Autodesk Fusion 360 part; units mm, degrees
(part 2 of 3)
  line L366 (210.5589, 31.2011) -> (210.5337, 34.6652)
  line L367 (213.9873, 40.7539) -> (210.9748, 42.464)
  line L368 (204.5338, 34.6214) -> (204.559, 31.1574)
  line L369 (201.0129, 37.1927) -> (204.0254, 35.4826)
  line L370 (210.9748, 42.464) -> (207.9875, 40.7102)
  line L371 (200.9877, 40.6567) -> (201.0129, 37.1927)
  line L372 (214.5714, 29.5007) -> (217.5587, 31.2545)
  line L373 (211.5336, 34.6749) -> (211.5588, 31.2108)
  line L374 (214.5209, 36.4287) -> (211.5336, 34.6749)
  line L375 (206.9875, 40.7005) -> (203.975, 42.4106)
  line L376 (207.5716, 29.4473) -> (210.5589, 31.2011)
  line L377 (210.5337, 34.6652) -> (207.5211, 36.3753)
  line L378 (207.9875, 40.7102) -> (208.0127, 37.2461)
  line L379 (204.0254, 35.4826) -> (207.0127, 37.2364)
  line L380 (211.5588, 31.2108) -> (214.5714, 29.5007)
  line L381 (207.5211, 36.3753) -> (204.5338, 34.6214)
  line L382 (208.0127, 37.2461) -> (211.0252, 35.536)
  line L383 (211.0252, 35.536) -> (214.0125, 37.2898)
  line L384 (207.0127, 37.2364) -> (206.9875, 40.7005)
  line L385 (203.975, 42.4106) -> (200.9877, 40.6567)
  line L386 (204.559, 31.1574) -> (207.5716, 29.4473)
  line L387 (214.0125, 37.2898) -> (213.9873, 40.7539)
  line L388 (217.5587, 31.2545) -> (217.5335, 34.7186)
  line L389 (217.5335, 34.7186) -> (214.5209, 36.4287)
  line L390 (224.5589, 31.2011) -> (224.5337, 34.6652)
  line L391 (227.9873, 40.7539) -> (224.9748, 42.464)
  line L392 (218.5338, 34.6214) -> (218.559, 31.1574)
  line L393 (215.0129, 37.1927) -> (218.0254, 35.4826)
  line L394 (224.9748, 42.464) -> (221.9875, 40.7102)
  line L395 (214.9877, 40.6567) -> (215.0129, 37.1927)
  line L396 (228.5714, 29.5007) -> (231.5587, 31.2545)
  line L397 (225.5336, 34.6749) -> (225.5588, 31.2108)
  line L398 (228.5209, 36.4287) -> (225.5336, 34.6749)
  line L399 (220.9875, 40.7005) -> (217.975, 42.4106)
  line L400 (221.5716, 29.4473) -> (224.5589, 31.2011)
  line L401 (224.5337, 34.6652) -> (221.5211, 36.3753)
  line L402 (221.9875, 40.7102) -> (222.0127, 37.2461)
  line L403 (218.0254, 35.4826) -> (221.0127, 37.2364)
  line L404 (225.5588, 31.2108) -> (228.5714, 29.5007)
  line L405 (221.5211, 36.3753) -> (218.5338, 34.6214)
  line L406 (222.0127, 37.2461) -> (225.0252, 35.536)
  line L407 (225.0252, 35.536) -> (228.0125, 37.2898)
  line L408 (221.0127, 37.2364) -> (220.9875, 40.7005)
  line L409 (217.975, 42.4106) -> (214.9877, 40.6567)
  line L410 (218.559, 31.1574) -> (221.5716, 29.4473)
  line L411 (228.0125, 37.2898) -> (227.9873, 40.7539)
  line L412 (231.5587, 31.2545) -> (231.5335, 34.7186)
  line L413 (231.5335, 34.7186) -> (228.5209, 36.4287)
  line L414 (140.5589, 43.2011) -> (140.5337, 46.6652)
  line L415 (143.9873, 52.7539) -> (140.9748, 54.464)
  line L416 (134.5338, 46.6214) -> (134.559, 43.1574)
  line L417 (131.0129, 49.1927) -> (134.0254, 47.4826)
  line L418 (140.9748, 54.464) -> (137.9875, 52.7102)
  line L419 (130.9877, 52.6567) -> (131.0129, 49.1927)
  line L420 (144.5714, 41.5007) -> (147.5587, 43.2545)
  line L421 (141.5336, 46.6749) -> (141.5588, 43.2108)
  line L422 (144.5209, 48.4287) -> (141.5336, 46.6749)
  line L423 (136.9875, 52.7005) -> (133.975, 54.4106)
  line L424 (137.5716, 41.4473) -> (140.5589, 43.2011)
  line L425 (140.5337, 46.6652) -> (137.5211, 48.3753)
  line L426 (137.9875, 52.7102) -> (138.0127, 49.2461)
  line L427 (134.0254, 47.4826) -> (137.0127, 49.2364)
  line L428 (141.5588, 43.2108) -> (144.5714, 41.5007)
  line L429 (137.5211, 48.3753) -> (134.5338, 46.6214)
  line L430 (138.0127, 49.2461) -> (141.0252, 47.536)
  line L431 (141.0252, 47.536) -> (144.0125, 49.2898)
  line L432 (137.0127, 49.2364) -> (136.9875, 52.7005)
  line L433 (133.975, 54.4106) -> (130.9877, 52.6567)
  line L434 (134.559, 43.1574) -> (137.5716, 41.4473)
  line L435 (144.0125, 49.2898) -> (143.9873, 52.7539)
  line L436 (147.5587, 43.2545) -> (147.5335, 46.7186)
  line L437 (147.5335, 46.7186) -> (144.5209, 48.4287)
  line L438 (154.5589, 43.2011) -> (154.5337, 46.6652)
  line L439 (157.9873, 52.7539) -> (154.9748, 54.464)
  line L440 (148.5338, 46.6214) -> (148.559, 43.1574)
  line L441 (145.0129, 49.1927) -> (148.0254, 47.4826)
  line L442 (154.9748, 54.464) -> (151.9875, 52.7102)
  line L443 (144.9877, 52.6567) -> (145.0129, 49.1927)
  line L444 (158.5714, 41.5007) -> (161.5587, 43.2545)
  line L445 (155.5336, 46.6749) -> (155.5588, 43.2108)
  line L446 (158.5209, 48.4287) -> (155.5336, 46.6749)
  line L447 (150.9875, 52.7005) -> (147.975, 54.4106)
  line L448 (151.5716, 41.4473) -> (154.5589, 43.2011)
  line L449 (154.5337, 46.6652) -> (151.5211, 48.3753)
  line L450 (151.9875, 52.7102) -> (152.0127, 49.2461)
  line L451 (148.0254, 47.4826) -> (151.0127, 49.2364)
  line L452 (155.5588, 43.2108) -> (158.5714, 41.5007)
  line L453 (151.5211, 48.3753) -> (148.5338, 46.6214)
  line L454 (152.0127, 49.2461) -> (155.0252, 47.536)
  line L455 (155.0252, 47.536) -> (158.0125, 49.2898)
  line L456 (151.0127, 49.2364) -> (150.9875, 52.7005)
  line L457 (147.975, 54.4106) -> (144.9877, 52.6567)
  line L458 (148.559, 43.1574) -> (151.5716, 41.4473)
  line L459 (158.0125, 49.2898) -> (157.9873, 52.7539)
  line L460 (161.5587, 43.2545) -> (161.5335, 46.7186)
  line L461 (161.5335, 46.7186) -> (158.5209, 48.4287)
  line L462 (168.5589, 43.2011) -> (168.5337, 46.6652)
  line L463 (171.9873, 52.7539) -> (168.9748, 54.464)
  line L464 (162.5338, 46.6214) -> (162.559, 43.1574)
  line L465 (159.0129, 49.1927) -> (162.0254, 47.4826)
  line L466 (168.9748, 54.464) -> (165.9875, 52.7102)
  line L467 (158.9877, 52.6567) -> (159.0129, 49.1927)
  line L468 (172.5714, 41.5007) -> (175.5587, 43.2545)
  line L469 (169.5336, 46.6749) -> (169.5588, 43.2108)
  line L470 (172.5209, 48.4287) -> (169.5336, 46.6749)
  line L471 (164.9875, 52.7005) -> (161.975, 54.4106)
  line L472 (165.5716, 41.4473) -> (168.5589, 43.2011)
  line L473 (168.5337, 46.6652) -> (165.5211, 48.3753)
  line L474 (165.9875, 52.7102) -> (166.0127, 49.2461)
  line L475 (162.0254, 47.4826) -> (165.0127, 49.2364)
  line L476 (169.5588, 43.2108) -> (172.5714, 41.5007)
  line L477 (165.5211, 48.3753) -> (162.5338, 46.6214)
  line L478 (166.0127, 49.2461) -> (169.0252, 47.536)
  line L479 (169.0252, 47.536) -> (172.0125, 49.2898)
  line L480 (165.0127, 49.2364) -> (164.9875, 52.7005)
  line L481 (161.975, 54.4106) -> (158.9877, 52.6567)
  line L482 (162.559, 43.1574) -> (165.5716, 41.4473)
  line L483 (172.0125, 49.2898) -> (171.9873, 52.7539)
  line L484 (175.5587, 43.2545) -> (175.5335, 46.7186)
  line L485 (175.5335, 46.7186) -> (172.5209, 48.4287)
  line L486 (182.5589, 43.2011) -> (182.5337, 46.6652)
  line L487 (185.9873, 52.7539) -> (182.9748, 54.464)
  line L488 (176.5338, 46.6214) -> (176.559, 43.1574)
  line L489 (173.0129, 49.1927) -> (176.0254, 47.4826)
  line L490 (182.9748, 54.464) -> (179.9875, 52.7102)
  line L491 (172.9877, 52.6567) -> (173.0129, 49.1927)
  line L492 (186.5714, 41.5007) -> (189.5587, 43.2545)
  line L493 (183.5336, 46.6749) -> (183.5588, 43.2108)
  line L494 (186.5209, 48.4287) -> (183.5336, 46.6749)
  line L495 (178.9875, 52.7005) -> (175.975, 54.4106)
  line L496 (179.5716, 41.4473) -> (182.5589, 43.2011)
  line L497 (182.5337, 46.6652) -> (179.5211, 48.3753)
  line L498 (179.9875, 52.7102) -> (180.0127, 49.2461)
  line L499 (176.0254, 47.4826) -> (179.0127, 49.2364)
  line L500 (183.5588, 43.2108) -> (186.5714, 41.5007)
  line L501 (179.5211, 48.3753) -> (176.5338, 46.6214)
  line L502 (180.0127, 49.2461) -> (183.0252, 47.536)
  line L503 (183.0252, 47.536) -> (186.0125, 49.2898)
  line L504 (179.0127, 49.2364) -> (178.9875, 52.7005)
  line L505 (175.975, 54.4106) -> (172.9877, 52.6567)
  line L506 (176.559, 43.1574) -> (179.5716, 41.4473)
  line L507 (186.0125, 49.2898) -> (185.9873, 52.7539)
  line L508 (189.5587, 43.2545) -> (189.5335, 46.7186)
  line L509 (189.5335, 46.7186) -> (186.5209, 48.4287)
  line L510 (196.5589, 43.2011) -> (196.5337, 46.6652)
  line L511 (199.9873, 52.7539) -> (196.9748, 54.464)
  line L512 (190.5338, 46.6214) -> (190.559, 43.1574)
  line L513 (187.0129, 49.1927) -> (190.0254, 47.4826)
  line L514 (196.9748, 54.464) -> (193.9875, 52.7102)
  line L515 (186.9877, 52.6567) -> (187.0129, 49.1927)
  line L516 (200.5714, 41.5007) -> (203.5587, 43.2545)
  line L517 (197.5336, 46.6749) -> (197.5588, 43.2108)
  line L518 (200.5209, 48.4287) -> (197.5336, 46.6749)
  line L519 (192.9875, 52.7005) -> (189.975, 54.4106)
  line L520 (193.5716, 41.4473) -> (196.5589, 43.2011)
  line L521 (196.5337, 46.6652) -> (193.5211, 48.3753)
  line L522 (193.9875, 52.7102) -> (194.0127, 49.2461)
  line L523 (190.0254, 47.4826) -> (193.0127, 49.2364)
  line L524 (197.5588, 43.2108) -> (200.5714, 41.5007)
  line L525 (193.5211, 48.3753) -> (190.5338, 46.6214)
  line L526 (194.0127, 49.2461) -> (197.0252, 47.536)
  line L527 (197.0252, 47.536) -> (200.0125, 49.2898)
  line L528 (193.0127, 49.2364) -> (192.9875, 52.7005)
  line L529 (189.975, 54.4106) -> (186.9877, 52.6567)
  line L530 (190.559, 43.1574) -> (193.5716, 41.4473)
  line L531 (200.0125, 49.2898) -> (199.9873, 52.7539)
  line L532 (203.5587, 43.2545) -> (203.5335, 46.7186)
  line L533 (203.5335, 46.7186) -> (200.5209, 48.4287)
  line L534 (210.5589, 43.2011) -> (210.5337, 46.6652)
  line L535 (213.9873, 52.7539) -> (210.9748, 54.464)
  line L536 (204.5338, 46.6214) -> (204.559, 43.1574)
  line L537 (201.0129, 49.1927) -> (204.0254, 47.4826)
  line L538 (210.9748, 54.464) -> (207.9875, 52.7102)
  line L539 (200.9877, 52.6567) -> (201.0129, 49.1927)
  line L540 (214.5714, 41.5007) -> (217.5587, 43.2545)
  line L541 (211.5336, 46.6749) -> (211.5588, 43.2108)
  line L542 (214.5209, 48.4287) -> (211.5336, 46.6749)
  line L543 (206.9875, 52.7005) -> (203.975, 54.4106)
  line L544 (207.5716, 41.4473) -> (210.5589, 43.2011)
  line L545 (210.5337, 46.6652) -> (207.5211, 48.3753)
  line L546 (207.9875, 52.7102) -> (208.0127, 49.2461)
  line L547 (204.0254, 47.4826) -> (207.0127, 49.2364)
  line L548 (211.5588, 43.2108) -> (214.5714, 41.5007)
  line L549 (207.5211, 48.3753) -> (204.5338, 46.6214)
  line L550 (208.0127, 49.2461) -> (211.0252, 47.536)
  line L551 (211.0252, 47.536) -> (214.0125, 49.2898)
  line L552 (207.0127, 49.2364) -> (206.9875, 52.7005)
  line L553 (203.975, 54.4106) -> (200.9877, 52.6567)
  line L554 (204.559, 43.1574) -> (207.5716, 41.4473)
  line L555 (214.0125, 49.2898) -> (213.9873, 52.7539)
  line L556 (217.5587, 43.2545) -> (217.5335, 46.7186)
  line L557 (217.5335, 46.7186) -> (214.5209, 48.4287)
  line L558 (224.5589, 43.2011) -> (224.5337, 46.6652)
  line L559 (227.9873, 52.7539) -> (224.9748, 54.464)
  line L560 (218.5338, 46.6214) -> (218.559, 43.1574)
  line L561 (215.0129, 49.1927) -> (218.0254, 47.4826)
  line L562 (224.9748, 54.464) -> (221.9875, 52.7102)
  line L563 (214.9877, 52.6567) -> (215.0129, 49.1927)
  line L564 (228.5714, 41.5007) -> (231.5587, 43.2545)
  line L565 (225.5336, 46.6749) -> (225.5588, 43.2108)
  line L566 (228.5209, 48.4287) -> (225.5336, 46.6749)
  line L567 (220.9875, 52.7005) -> (217.975, 54.4106)
  line L568 (221.5716, 41.4473) -> (224.5589, 43.2011)
  line L569 (224.5337, 46.6652) -> (221.5211, 48.3753)
  line L570 (221.9875, 52.7102) -> (222.0127, 49.2461)
  line L571 (218.0254, 47.4826) -> (221.0127, 49.2364)
  line L572 (225.5588, 43.2108) -> (228.5714, 41.5007)
  line L573 (221.5211, 48.3753) -> (218.5338, 46.6214)
  line L574 (222.0127, 49.2461) -> (225.0252, 47.536)
  line L575 (225.0252, 47.536) -> (228.0125, 49.2898)
  line L576 (221.0127, 49.2364) -> (220.9875, 52.7005)
  line L577 (217.975, 54.4106) -> (214.9877, 52.6567)
  line L578 (218.559, 43.1574) -> (221.5716, 41.4473)
  line L579 (228.0125, 49.2898) -> (227.9873, 52.7539)
  line L580 (231.5587, 43.2545) -> (231.5335, 46.7186)
  line L581 (231.5335, 46.7186) -> (228.5209, 48.4287)
  line L582 (140.5589, 55.2011) -> (140.5337, 58.6652)
  line L583 (143.9873, 64.7539) -> (140.9748, 66.464)
  line L584 (134.5338, 58.6214) -> (134.559, 55.1574)
  line L585 (131.0129, 61.1927) -> (134.0254, 59.4826)
  line L586 (140.9748, 66.464) -> (137.9875, 64.7102)
  line L587 (130.9877, 64.6567) -> (131.0129, 61.1927)
  line L588 (144.5714, 53.5007) -> (147.5587, 55.2545)
  line L589 (141.5336, 58.6749) -> (141.5588, 55.2108)
  line L590 (144.5209, 60.4287) -> (141.5336, 58.6749)
  line L591 (136.9875, 64.7005) -> (133.975, 66.4106)
  line L592 (137.5716, 53.4473) -> (140.5589, 55.2011)
  line L593 (140.5337, 58.6652) -> (137.5211, 60.3753)
  line L594 (137.9875, 64.7102) -> (138.0127, 61.2461)
  line L595 (134.0254, 59.4826) -> (137.0127, 61.2364)
  line L596 (141.5588, 55.2108) -> (144.5714, 53.5007)
  line L597 (137.5211, 60.3753) -> (134.5338, 58.6214)
  line L598 (138.0127, 61.2461) -> (141.0252, 59.536)
  line L599 (141.0252, 59.536) -> (144.0125, 61.2898)
  line L600 (137.0127, 61.2364) -> (136.9875, 64.7005)
  line L601 (133.975, 66.4106) -> (130.9877, 64.6567)
  line L602 (134.559, 55.1574) -> (137.5716, 53.4473)
  line L603 (144.0125, 61.2898) -> (143.9873, 64.7539)
  line L604 (147.5587, 55.2545) -> (147.5335, 58.7186)
  line L605 (147.5335, 58.7186) -> (144.5209, 60.4287)
  line L606 (154.5589, 55.2011) -> (154.5337, 58.6652)
  line L607 (157.9873, 64.7539) -> (154.9748, 66.464)
  line L608 (148.5338, 58.6214) -> (148.559, 55.1574)
  line L609 (145.0129, 61.1927) -> (148.0254, 59.4826)
  line L610 (154.9748, 66.464) -> (151.9875, 64.7102)
  line L611 (144.9877, 64.6567) -> (145.0129, 61.1927)
  line L612 (158.5714, 53.5007) -> (161.5587, 55.2545)
  line L613 (155.5336, 58.6749) -> (155.5588, 55.2108)
  line L614 (158.5209, 60.4287) -> (155.5336, 58.6749)
  line L615 (150.9875, 64.7005) -> (147.975, 66.4106)
  line L616 (151.5716, 53.4473) -> (154.5589, 55.2011)
  line L617 (154.5337, 58.6652) -> (151.5211, 60.3753)
  line L618 (151.9875, 64.7102) -> (152.0127, 61.2461)
  line L619 (148.0254, 59.4826) -> (151.0127, 61.2364)
  line L620 (155.5588, 55.2108) -> (158.5714, 53.5007)
  line L621 (151.5211, 60.3753) -> (148.5338, 58.6214)
  line L622 (152.0127, 61.2461) -> (155.0252, 59.536)
  line L623 (155.0252, 59.536) -> (158.0125, 61.2898)
  line L624 (151.0127, 61.2364) -> (150.9875, 64.7005)
  line L625 (147.975, 66.4106) -> (144.9877, 64.6567)
  line L626 (148.559, 55.1574) -> (151.5716, 53.4473)
  line L627 (158.0125, 61.2898) -> (157.9873, 64.7539)
  line L628 (161.5587, 55.2545) -> (161.5335, 58.7186)
  line L629 (161.5335, 58.7186) -> (158.5209, 60.4287)
  line L630 (168.5589, 55.2011) -> (168.5337, 58.6652)
  line L631 (171.9873, 64.7539) -> (168.9748, 66.464)
  line L632 (162.5338, 58.6214) -> (162.559, 55.1574)
  line L633 (159.0129, 61.1927) -> (162.0254, 59.4826)
  line L634 (168.9748, 66.464) -> (165.9875, 64.7102)
  line L635 (158.9877, 64.6567) -> (159.0129, 61.1927)
  line L636 (172.5714, 53.5007) -> (175.5587, 55.2545)
  line L637 (169.5336, 58.6749) -> (169.5588, 55.2108)
  line L638 (172.5209, 60.4287) -> (169.5336, 58.6749)
  line L639 (164.9875, 64.7005) -> (161.975, 66.4106)
  line L640 (165.5716, 53.4473) -> (168.5589, 55.2011)
  line L641 (168.5337, 58.6652) -> (165.5211, 60.3753)
  line L642 (165.9875, 64.7102) -> (166.0127, 61.2461)
  line L643 (162.0254, 59.4826) -> (165.0127, 61.2364)
  line L644 (169.5588, 55.2108) -> (172.5714, 53.5007)
  line L645 (165.5211, 60.3753) -> (162.5338, 58.6214)
  line L646 (166.0127, 61.2461) -> (169.0252, 59.536)
  line L647 (169.0252, 59.536) -> (172.0125, 61.2898)
  line L648 (165.0127, 61.2364) -> (164.9875, 64.7005)
  line L649 (161.975, 66.4106) -> (158.9877, 64.6567)
  line L650 (162.559, 55.1574) -> (165.5716, 53.4473)
  line L651 (172.0125, 61.2898) -> (171.9873, 64.7539)
  line L652 (175.5587, 55.2545) -> (175.5335, 58.7186)
  line L653 (175.5335, 58.7186) -> (172.5209, 60.4287)
  line L654 (196.5589, 55.2011) -> (196.5337, 58.6652)
  line L655 (199.9873, 64.7539) -> (196.9748, 66.464)
  line L656 (190.5338, 58.6214) -> (190.559, 55.1574)
  line L657 (187.0129, 61.1927) -> (190.0254, 59.4826)
  line L658 (196.9748, 66.464) -> (193.9875, 64.7102)
  line L659 (186.9877, 64.6567) -> (187.0129, 61.1927)
  line L660 (200.5714, 53.5007) -> (203.5587, 55.2545)
  line L661 (197.5336, 58.6749) -> (197.5588, 55.2108)
  line L662 (200.5209, 60.4287) -> (197.5336, 58.6749)
  line L663 (192.9875, 64.7005) -> (189.975, 66.4106)
  line L664 (193.5716, 53.4473) -> (196.5589, 55.2011)
  line L665 (196.5337, 58.6652) -> (193.5211, 60.3753)
  line L666 (193.9875, 64.7102) -> (194.0127, 61.2461)
  line L667 (190.0254, 59.4826) -> (193.0127, 61.2364)
  line L668 (197.5588, 55.2108) -> (200.5714, 53.5007)
  line L669 (193.5211, 60.3753) -> (190.5338, 58.6214)
  line L670 (194.0127, 61.2461) -> (197.0252, 59.536)
  line L671 (197.0252, 59.536) -> (200.0125, 61.2898)
  line L672 (193.0127, 61.2364) -> (192.9875, 64.7005)
  line L673 (189.975, 66.4106) -> (186.9877, 64.6567)
  line L674 (190.559, 55.1574) -> (193.5716, 53.4473)
  line L675 (200.0125, 61.2898) -> (199.9873, 64.7539)
  line L676 (203.5587, 55.2545) -> (203.5335, 58.7186)
  line L677 (203.5335, 58.7186) -> (200.5209, 60.4287)
  line L678 (210.5589, 55.2011) -> (210.5337, 58.6652)
  line L679 (213.9873, 64.7539) -> (210.9748, 66.464)
  line L680 (204.5338, 58.6214) -> (204.559, 55.1574)
  line L681 (201.0129, 61.1927) -> (204.0254, 59.4826)
  line L682 (210.9748, 66.464) -> (207.9875, 64.7102)
  line L683 (200.9877, 64.6567) -> (201.0129, 61.1927)
  line L684 (214.5714, 53.5007) -> (217.5587, 55.2545)
  line L685 (211.5336, 58.6749) -> (211.5588, 55.2108)
  line L686 (214.5209, 60.4287) -> (211.5336, 58.6749)
  line L687 (206.9875, 64.7005) -> (203.975, 66.4106)
  line L688 (207.5716, 53.4473) -> (210.5589, 55.2011)
  line L689 (210.5337, 58.6652) -> (207.5211, 60.3753)
  line L690 (207.9875, 64.7102) -> (208.0127, 61.2461)
  line L691 (204.0254, 59.4826) -> (207.0127, 61.2364)
  line L692 (211.5588, 55.2108) -> (214.5714, 53.5007)
  line L693 (207.5211, 60.3753) -> (204.5338, 58.6214)
  line L694 (208.0127, 61.2461) -> (211.0252, 59.536)
  line L695 (211.0252, 59.536) -> (214.0125, 61.2898)
  line L696 (207.0127, 61.2364) -> (206.9875, 64.7005)
  line L697 (203.975, 66.4106) -> (200.9877, 64.6567)
  line L698 (204.559, 55.1574) -> (207.5716, 53.4473)
  line L699 (214.0125, 61.2898) -> (213.9873, 64.7539)
  line L700 (217.5587, 55.2545) -> (217.5335, 58.7186)
  line L701 (217.5335, 58.7186) -> (214.5209, 60.4287)
  line L702 (224.5589, 55.2011) -> (224.5337, 58.6652)
  line L703 (227.9873, 64.7539) -> (224.9748, 66.464)
  line L704 (218.5338, 58.6214) -> (218.559, 55.1574)
  line L705 (215.0129, 61.1927) -> (218.0254, 59.4826)
  line L706 (224.9748, 66.464) -> (221.9875, 64.7102)
  line L707 (214.9877, 64.6567) -> (215.0129, 61.1927)
  line L708 (228.5714, 53.5007) -> (231.5587, 55.2545)
  line L709 (225.5336, 58.6749) -> (225.5588, 55.2108)
  line L710 (228.5209, 60.4287) -> (225.5336, 58.6749)
  line L711 (220.9875, 64.7005) -> (217.975, 66.4106)
  line L712 (221.5716, 53.4473) -> (224.5589, 55.2011)
  line L713 (224.5337, 58.6652) -> (221.5211, 60.3753)
  line L714 (221.9875, 64.7102) -> (222.0127, 61.2461)
  line L715 (218.0254, 59.4826) -> (221.0127, 61.2364)
  line L716 (225.5588, 55.2108) -> (228.5714, 53.5007)
  line L717 (221.5211, 60.3753) -> (218.5338, 58.6214)
  line L718 (222.0127, 61.2461) -> (225.0252, 59.536)
  line L719 (225.0252, 59.536) -> (228.0125, 61.2898)
  line L720 (221.0127, 61.2364) -> (220.9875, 64.7005)
  line L721 (217.975, 66.4106) -> (214.9877, 64.6567)
  line L722 (218.559, 55.1574) -> (221.5716, 53.4473)
  line L723 (228.0125, 61.2898) -> (227.9873, 64.7539)
  line L724 (231.5587, 55.2545) -> (231.5335, 58.7186)
  line L725 (231.5335, 58.7186) -> (228.5209, 60.4287)
  line L726 (140.5589, 67.2011) -> (140.5337, 70.6652)
  line L727 (143.9873, 76.7539) -> (140.9748, 78.464)
  line L728 (134.5338, 70.6214) -> (134.559, 67.1574)
  line L729 (131.0129, 73.1927) -> (134.0254, 71.4826)
  line L730 (140.9748, 78.464) -> (137.9875, 76.7102)
  line L731 (130.9877, 76.6567) -> (131.0129, 73.1927)
  line L732 (144.5714, 65.5007) -> (147.5587, 67.2545)
  line L733 (141.5336, 70.6749) -> (141.5588, 67.2108)
  line L734 (144.5209, 72.4287) -> (141.5336, 70.6749)
  line L735 (136.9875, 76.7005) -> (133.975, 78.4106)
  line L736 (137.5716, 65.4473) -> (140.5589, 67.2011)
  line L737 (140.5337, 70.6652) -> (137.5211, 72.3753)
  line L738 (137.9875, 76.7102) -> (138.0127, 73.2461)
  line L739 (134.0254, 71.4826) -> (137.0127, 73.2364)
  line L740 (141.5588, 67.2108) -> (144.5714, 65.5007)
  line L741 (137.5211, 72.3753) -> (134.5338, 70.6214)
  line L742 (138.0127, 73.2461) -> (141.0252, 71.536)
  line L743 (141.0252, 71.536) -> (144.0125, 73.2898)
  line L744 (137.0127, 73.2364) -> (136.9875, 76.7005)
  line L745 (133.975, 78.4106) -> (130.9877, 76.6567)
  line L746 (134.559, 67.1574) -> (137.5716, 65.4473)
  line L747 (144.0125, 73.2898) -> (143.9873, 76.7539)
  line L748 (147.5587, 67.2545) -> (147.5335, 70.7186)
  line L749 (147.5335, 70.7186) -> (144.5209, 72.4287)
  line L750 (154.5589, 67.2011) -> (154.5337, 70.6652)
  line L751 (157.9873, 76.7539) -> (154.9748, 78.464)
  line L752 (148.5338, 70.6214) -> (148.559, 67.1574)
  line L753 (145.0129, 73.1927) -> (148.0254, 71.4826)
  line L754 (154.9748, 78.464) -> (151.9875, 76.7102)
  line L755 (144.9877, 76.6567) -> (145.0129, 73.1927)
  line L756 (158.5714, 65.5007) -> (161.5587, 67.2545)
  line L757 (155.5336, 70.6749) -> (155.5588, 67.2108)
  line L758 (158.5209, 72.4287) -> (155.5336, 70.6749)
  line L759 (150.9875, 76.7005) -> (147.975, 78.4106)
  line L760 (151.5716, 65.4473) -> (154.5589, 67.2011)
  line L761 (154.5337, 70.6652) -> (151.5211, 72.3753)
  line L762 (151.9875, 76.7102) -> (152.0127, 73.2461)
  line L763 (148.0254, 71.4826) -> (151.0127, 73.2364)
  line L764 (155.5588, 67.2108) -> (158.5714, 65.5007)
  line L765 (151.5211, 72.3753) -> (148.5338, 70.6214)
  line L766 (152.0127, 73.2461) -> (155.0252, 71.536)
  line L767 (155.0252, 71.536) -> (158.0125, 73.2898)
  line L768 (151.0127, 73.2364) -> (150.9875, 76.7005)
  line L769 (147.975, 78.4106) -> (144.9877, 76.6567)
  line L770 (148.559, 67.1574) -> (151.5716, 65.4473)
  line L771 (158.0125, 73.2898) -> (157.9873, 76.7539)
  line L772 (161.5587, 67.2545) -> (161.5335, 70.7186)
  line L773 (161.5335, 70.7186) -> (158.5209, 72.4287)
  line L774 (168.5589, 67.2011) -> (168.5337, 70.6652)
  line L775 (171.9873, 76.7539) -> (168.9748, 78.464)
  line L776 (162.5338, 70.6214) -> (162.559, 67.1574)
  line L777 (159.0129, 73.1927) -> (162.0254, 71.4826)
  line L778 (168.9748, 78.464) -> (165.9875, 76.7102)
  line L779 (158.9877, 76.6567) -> (159.0129, 73.1927)
  line L780 (172.5714, 65.5007) -> (175.5587, 67.2545)
  line L781 (169.5336, 70.6749) -> (169.5588, 67.2108)
  line L782 (172.5209, 72.4287) -> (169.5336, 70.6749)
  line L783 (164.9875, 76.7005) -> (161.975, 78.4106)
  line L784 (165.5716, 65.4473) -> (168.5589, 67.2011)
  line L785 (168.5337, 70.6652) -> (165.5211, 72.3753)
  line L786 (165.9875, 76.7102) -> (166.0127, 73.2461)
  line L787 (162.0254, 71.4826) -> (165.0127, 73.2364)
  line L788 (169.5588, 67.2108) -> (172.5714, 65.5007)
  line L789 (165.5211, 72.3753) -> (162.5338, 70.6214)
  line L790 (166.0127, 73.2461) -> (169.0252, 71.536)
  line L791 (169.0252, 71.536) -> (172.0125, 73.2898)
  line L792 (165.0127, 73.2364) -> (164.9875, 76.7005)
  line L793 (161.975, 78.4106) -> (158.9877, 76.6567)
  line L794 (162.559, 67.1574) -> (165.5716, 65.4473)
  line L795 (172.0125, 73.2898) -> (171.9873, 76.7539)
  line L796 (175.5587, 67.2545) -> (175.5335, 70.7186)
  line L797 (175.5335, 70.7186) -> (172.5209, 72.4287)
  line L798 (182.5589, 67.2011) -> (182.5337, 70.6652)
  line L799 (185.9873, 76.7539) -> (182.9748, 78.464)
  line L800 (176.5338, 70.6214) -> (176.559, 67.1574)
  line L801 (173.0129, 73.1927) -> (176.0254, 71.4826)
  line L802 (182.9748, 78.464) -> (179.9875, 76.7102)
  line L803 (172.9877, 76.6567) -> (173.0129, 73.1927)
  line L804 (186.5714, 65.5007) -> (189.5587, 67.2545)
  line L805 (183.5336, 70.6749) -> (183.5588, 67.2108)
  line L806 (186.5209, 72.4287) -> (183.5336, 70.6749)
  line L807 (178.9875, 76.7005) -> (175.975, 78.4106)
  line L808 (179.5716, 65.4473) -> (182.5589, 67.2011)
  line L809 (182.5337, 70.6652) -> (179.5211, 72.3753)
  line L810 (179.9875, 76.7102) -> (180.0127, 73.2461)
  line L811 (176.0254, 71.4826) -> (179.0127, 73.2364)
  line L812 (183.5588, 67.2108) -> (186.5714, 65.5007)
  line L813 (179.5211, 72.3753) -> (176.5338, 70.6214)
  line L814 (180.0127, 73.2461) -> (183.0252, 71.536)
  line L815 (183.0252, 71.536) -> (186.0125, 73.2898)
  line L816 (179.0127, 73.2364) -> (178.9875, 76.7005)
  line L817 (175.975, 78.4106) -> (172.9877, 76.6567)
  line L818 (176.559, 67.1574) -> (179.5716, 65.4473)
  line L819 (186.0125, 73.2898) -> (185.9873, 76.7539)
  line L820 (189.5587, 67.2545) -> (189.5335, 70.7186)
  line L821 (189.5335, 70.7186) -> (186.5209, 72.4287)
  line L822 (196.5589, 67.2011) -> (196.5337, 70.6652)
  line L823 (199.9873, 76.7539) -> (196.9748, 78.464)
  line L824 (190.5338, 70.6214) -> (190.559, 67.1574)
  line L825 (187.0129, 73.1927) -> (190.0254, 71.4826)
  line L826 (196.9748, 78.464) -> (193.9875, 76.7102)
  line L827 (186.9877, 76.6567) -> (187.0129, 73.1927)
  line L828 (200.5714, 65.5007) -> (203.5587, 67.2545)
  line L829 (197.5336, 70.6749) -> (197.5588, 67.2108)
  line L830 (200.5209, 72.4287) -> (197.5336, 70.6749)
  line L831 (192.9875, 76.7005) -> (189.975, 78.4106)
  line L832 (193.5716, 65.4473) -> (196.5589, 67.2011)
  line L833 (196.5337, 70.6652) -> (193.5211, 72.3753)
  line L834 (193.9875, 76.7102) -> (194.0127, 73.2461)
  line L835 (190.0254, 71.4826) -> (193.0127, 73.2364)
  line L836 (197.5588, 67.2108) -> (200.5714, 65.5007)
  line L837 (193.5211, 72.3753) -> (190.5338, 70.6214)
  line L838 (194.0127, 73.2461) -> (197.0252, 71.536)
  line L839 (197.0252, 71.536) -> (200.0125, 73.2898)
  line L840 (193.0127, 73.2364) -> (192.9875, 76.7005)
  line L841 (189.975, 78.4106) -> (186.9877, 76.6567)
  line L842 (190.559, 67.1574) -> (193.5716, 65.4473)
  line L843 (200.0125, 73.2898) -> (199.9873, 76.7539)
  line L844 (203.5587, 67.2545) -> (203.5335, 70.7186)
  line L845 (203.5335, 70.7186) -> (200.5209, 72.4287)
  line L846 (210.5589, 67.2011) -> (210.5337, 70.6652)
  line L847 (213.9873, 76.7539) -> (210.9748, 78.464)
  line L848 (204.5338, 70.6214) -> (204.559, 67.1574)
  line L849 (201.0129, 73.1927) -> (204.0254, 71.4826)
  line L850 (210.9748, 78.464) -> (207.9875, 76.7102)
  line L851 (200.9877, 76.6567) -> (201.0129, 73.1927)
  line L852 (214.5714, 65.5007) -> (217.5587, 67.2545)
  line L853 (211.5336, 70.6749) -> (211.5588, 67.2108)
  line L854 (214.5209, 72.4287) -> (211.5336, 70.6749)
  line L855 (206.9875, 76.7005) -> (203.975, 78.4106)
  line L856 (207.5716, 65.4473) -> (210.5589, 67.2011)
  line L857 (210.5337, 70.6652) -> (207.5211, 72.3753)
  line L858 (207.9875, 76.7102) -> (208.0127, 73.2461)
  line L859 (204.0254, 71.4826) -> (207.0127, 73.2364)
  line L860 (211.5588, 67.2108) -> (214.5714, 65.5007)
  line L861 (207.5211, 72.3753) -> (204.5338, 70.6214)
  line L862 (208.0127, 73.2461) -> (211.0252, 71.536)
  line L863 (211.0252, 71.536) -> (214.0125, 73.2898)
  line L864 (207.0127, 73.2364) -> (206.9875, 76.7005)
  line L865 (203.975, 78.4106) -> (200.9877, 76.6567)
  line L866 (204.559, 67.1574) -> (207.5716, 65.4473)
  line L867 (214.0125, 73.2898) -> (213.9873, 76.7539)
  line L868 (217.5587, 67.2545) -> (217.5335, 70.7186)
  line L869 (217.5335, 70.7186) -> (214.5209, 72.4287)
  line L870 (224.5589, 67.2011) -> (224.5337, 70.6652)
  line L871 (227.9873, 76.7539) -> (224.9748, 78.464)
  line L872 (218.5338, 70.6214) -> (218.559, 67.1574)
  line L873 (215.0129, 73.1927) -> (218.0254, 71.4826)
  line L874 (224.9748, 78.464) -> (221.9875, 76.7102)
  line L875 (214.9877, 76.6567) -> (215.0129, 73.1927)
  line L876 (228.5714, 65.5007) -> (231.5587, 67.2545)
  line L877 (225.5336, 70.6749) -> (225.5588, 67.2108)
  line L878 (228.5209, 72.4287) -> (225.5336, 70.6749)
  line L879 (220.9875, 76.7005) -> (217.975, 78.4106)
  line L880 (221.5716, 65.4473) -> (224.5589, 67.2011)
  line L881 (224.5337, 70.6652) -> (221.5211, 72.3753)
  line L882 (221.9875, 76.7102) -> (222.0127, 73.2461)
  line L883 (218.0254, 71.4826) -> (221.0127, 73.2364)
  line L884 (225.5588, 67.2108) -> (228.5714, 65.5007)
  line L885 (221.5211, 72.3753) -> (218.5338, 70.6214)
  line L886 (222.0127, 73.2461) -> (225.0252, 71.536)
  line L887 (225.0252, 71.536) -> (228.0125, 73.2898)
  line L888 (221.0127, 73.2364) -> (220.9875, 76.7005)
  line L889 (217.975, 78.4106) -> (214.9877, 76.6567)
  line L890 (218.559, 67.1574) -> (221.5716, 65.4473)
  line L891 (228.0125, 73.2898) -> (227.9873, 76.7539)
  line L892 (231.5587, 67.2545) -> (231.5335, 70.7186)
  line L893 (231.5335, 70.7186) -> (228.5209, 72.4287)
  line L894 (140.5589, 79.2011) -> (140.5337, 82.6652)
  line L895 (134.5338, 82.6214) -> (134.559, 79.1574)
  line L896 (131.0129, 85.1927) -> (134.0254, 83.4826)
  line L897 (140.9748, 90.464) -> (137.9875, 88.7102)
  line L898 (130.9877, 88.6567) -> (131.0129, 85.1927)
  line L899 (144.5714, 77.5007) -> (147.5587, 79.2545)
  line L900 (141.5336, 82.6749) -> (141.5588, 79.2108)
  line L901 (136.9875, 88.7005) -> (133.975, 90.4106)
  line L902 (137.5716, 77.4473) -> (140.5589, 79.2011)
  line L903 (140.5337, 82.6652) -> (137.5211, 84.3753)
  line L904 (137.9875, 88.7102) -> (138.0127, 85.2461)
  line L905 (134.0254, 83.4826) -> (137.0127, 85.2364)
  line L906 (141.5588, 79.2108) -> (144.5714, 77.5007)
  line L907 (137.5211, 84.3753) -> (134.5338, 82.6214)
  line L908 (137.0127, 85.2364) -> (136.9875, 88.7005)
  line L909 (133.975, 90.4106) -> (130.9877, 88.6567)
  line L910 (134.559, 79.1574) -> (137.5716, 77.4473)
  line L911 (147.5587, 79.2545) -> (147.5335, 82.7186)
  line L912 (147.5335, 82.7186) -> (144.5209, 84.4287)
  line L913 (154.5589, 79.2011) -> (154.5337, 82.6652)
  line L914 (157.9873, 88.7539) -> (154.9748, 90.464)
  line L915 (148.5338, 82.6214) -> (148.559, 79.1574)
  line L916 (145.0129, 85.1927) -> (148.0254, 83.4826)
  line L917 (154.9748, 90.464) -> (151.9875, 88.7102)
  line L918 (158.5714, 77.5007) -> (161.5587, 79.2545)
  line L919 (155.5336, 82.6749) -> (155.5588, 79.2108)
  line L920 (158.5209, 84.4287) -> (155.5336, 82.6749)
  line L921 (150.9875, 88.7005) -> (147.975, 90.4106)
  line L922 (151.5716, 77.4473) -> (154.5589, 79.2011)
  line L923 (154.5337, 82.6652) -> (151.5211, 84.3753)
  line L924 (151.9875, 88.7102) -> (152.0127, 85.2461)
  line L925 (148.0254, 83.4826) -> (151.0127, 85.2364)
  line L926 (155.5588, 79.2108) -> (158.5714, 77.5007)
  line L927 (151.5211, 84.3753) -> (148.5338, 82.6214)
  line L928 (152.0127, 85.2461) -> (155.0252, 83.536)
  line L929 (155.0252, 83.536) -> (158.0125, 85.2898)
  line L930 (151.0127, 85.2364) -> (150.9875, 88.7005)
  line L931 (147.975, 90.4106) -> (144.9877, 88.6567)
  line L932 (148.559, 79.1574) -> (151.5716, 77.4473)
  line L933 (158.0125, 85.2898) -> (157.9873, 88.7539)
  line L934 (161.5587, 79.2545) -> (161.5335, 82.7186)
  line L935 (161.5335, 82.7186) -> (158.5209, 84.4287)
  line L936 (168.5589, 79.2011) -> (168.5337, 82.6652)
  line L937 (171.9873, 88.7539) -> (168.9748, 90.464)
  line L938 (162.5338, 82.6214) -> (162.559, 79.1574)
  line L939 (159.0129, 85.1927) -> (162.0254, 83.4826)
  line L940 (168.9748, 90.464) -> (165.9875, 88.7102)
  line L941 (158.9877, 88.6567) -> (159.0129, 85.1927)
  line L942 (172.5714, 77.5007) -> (175.5587, 79.2545)
  line L943 (169.5336, 82.6749) -> (169.5588, 79.2108)
  line L944 (172.5209, 84.4287) -> (169.5336, 82.6749)
  line L945 (164.9875, 88.7005) -> (161.975, 90.4106)
  line L946 (165.5716, 77.4473) -> (168.5589, 79.2011)
  line L947 (168.5337, 82.6652) -> (165.5211, 84.3753)
  line L948 (165.9875, 88.7102) -> (166.0127, 85.2461)
  line L949 (162.0254, 83.4826) -> (165.0127, 85.2364)
  line L950 (169.5588, 79.2108) -> (172.5714, 77.5007)
  line L951 (165.5211, 84.3753) -> (162.5338, 82.6214)
  line L952 (166.0127, 85.2461) -> (169.0252, 83.536)
  line L953 (169.0252, 83.536) -> (172.0125, 85.2898)
  line L954 (165.0127, 85.2364) -> (164.9875, 88.7005)
  line L955 (161.975, 90.4106) -> (158.9877, 88.6567)
  line L956 (162.559, 79.1574) -> (165.5716, 77.4473)
  line L957 (172.0125, 85.2898) -> (171.9873, 88.7539)
  line L958 (175.5587, 79.2545) -> (175.5335, 82.7186)
  line L959 (175.5335, 82.7186) -> (172.5209, 84.4287)
  line L960 (182.5589, 79.2011) -> (182.5337, 82.6652)
  line L961 (185.9873, 88.7539) -> (182.9748, 90.464)
  line L962 (176.5338, 82.6214) -> (176.559, 79.1574)
  line L963 (173.0129, 85.1927) -> (176.0254, 83.4826)
  line L964 (182.9748, 90.464) -> (179.9875, 88.7102)
  line L965 (172.9877, 88.6567) -> (173.0129, 85.1927)
  line L966 (186.5714, 77.5007) -> (189.5587, 79.2545)
  line L967 (183.5336, 82.6749) -> (183.5588, 79.2108)
  line L968 (186.5209, 84.4287) -> (183.5336, 82.6749)
  line L969 (178.9875, 88.7005) -> (175.975, 90.4106)
  line L970 (179.5716, 77.4473) -> (182.5589, 79.2011)
  line L971 (182.5337, 82.6652) -> (179.5211, 84.3753)
  line L972 (179.9875, 88.7102) -> (180.0127, 85.2461)
  line L973 (176.0254, 83.4826) -> (179.0127, 85.2364)
  line L974 (183.5588, 79.2108) -> (186.5714, 77.5007)
  line L975 (179.5211, 84.3753) -> (176.5338, 82.6214)
  line L976 (180.0127, 85.2461) -> (183.0252, 83.536)
  line L977 (183.0252, 83.536) -> (186.0125, 85.2898)
  line L978 (179.0127, 85.2364) -> (178.9875, 88.7005)
  line L979 (175.975, 90.4106) -> (172.9877, 88.6567)
  line L980 (176.559, 79.1574) -> (179.5716, 77.4473)
  line L981 (186.0125, 85.2898) -> (185.9873, 88.7539)
  line L982 (189.5587, 79.2545) -> (189.5335, 82.7186)
  line L983 (189.5335, 82.7186) -> (186.5209, 84.4287)
  line L984 (196.5589, 79.2011) -> (196.5337, 82.6652)
  line L985 (199.9873, 88.7539) -> (196.9748, 90.464)
  line L986 (190.5338, 82.6214) -> (190.559, 79.1574)
  line L987 (187.0129, 85.1927) -> (190.0254, 83.4826)
  line L988 (196.9748, 90.464) -> (193.9875, 88.7102)
  line L989 (186.9877, 88.6567) -> (187.0129, 85.1927)
  line L990 (200.5714, 77.5007) -> (203.5587, 79.2545)
  line L991 (197.5336, 82.6749) -> (197.5588, 79.2108)
  line L992 (200.5209, 84.4287) -> (197.5336, 82.6749)
  line L993 (192.9875, 88.7005) -> (189.975, 90.4106)
  line L994 (193.5716, 77.4473) -> (196.5589, 79.2011)
  line L995 (196.5337, 82.6652) -> (193.5211, 84.3753)
  line L996 (193.9875, 88.7102) -> (194.0127, 85.2461)
  line L997 (190.0254, 83.4826) -> (193.0127, 85.2364)
  line L998 (197.5588, 79.2108) -> (200.5714, 77.5007)
  line L999 (193.5211, 84.3753) -> (190.5338, 82.6214)
  line L1000 (194.0127, 85.2461) -> (197.0252, 83.536)
  line L1001 (197.0252, 83.536) -> (200.0125, 85.2898)
  line L1002 (193.0127, 85.2364) -> (192.9875, 88.7005)
  line L1003 (189.975, 90.4106) -> (186.9877, 88.6567)
  line L1004 (190.559, 79.1574) -> (193.5716, 77.4473)
  line L1005 (200.0125, 85.2898) -> (199.9873, 88.7539)
  line L1006 (203.5587, 79.2545) -> (203.5335, 82.7186)
  line L1007 (203.5335, 82.7186) -> (200.5209, 84.4287)
  line L1008 (210.5589, 79.2011) -> (210.5337, 82.6652)
  line L1009 (213.9873, 88.7539) -> (210.9748, 90.464)
  line L1010 (204.5338, 82.6214) -> (204.559, 79.1574)
  line L1011 (201.0129, 85.1927) -> (204.0254, 83.4826)
  line L1012 (210.9748, 90.464) -> (207.9875, 88.7102)
  line L1013 (200.9877, 88.6567) -> (201.0129, 85.1927)
  line L1014 (214.5714, 77.5007) -> (217.5587, 79.2545)
  line L1015 (211.5336, 82.6749) -> (211.5588, 79.2108)
  line L1016 (214.5209, 84.4287) -> (211.5336, 82.6749)
  line L1017 (206.9875, 88.7005) -> (203.975, 90.4106)
  line L1018 (207.5716, 77.4473) -> (210.5589, 79.2011)
  line L1019 (210.5337, 82.6652) -> (207.5211, 84.3753)
  line L1020 (207.9875, 88.7102) -> (208.0127, 85.2461)
  line L1021 (204.0254, 83.4826) -> (207.0127, 85.2364)
  line L1022 (211.5588, 79.2108) -> (214.5714, 77.5007)
  line L1023 (207.5211, 84.3753) -> (204.5338, 82.6214)
  line L1024 (208.0127, 85.2461) -> (211.0252, 83.536)
  line L1025 (211.0252, 83.536) -> (214.0125, 85.2898)
  line L1026 (207.0127, 85.2364) -> (206.9875, 88.7005)
  line L1027 (203.975, 90.4106) -> (200.9877, 88.6567)
  line L1028 (204.559, 79.1574) -> (207.5716, 77.4473)
  line L1029 (214.0125, 85.2898) -> (213.9873, 88.7539)
  line L1030 (217.5587, 79.2545) -> (217.5335, 82.7186)
  line L1031 (217.5335, 82.7186) -> (214.5209, 84.4287)
  line L1032 (224.5589, 79.2011) -> (224.5337, 82.6652)
  line L1033 (227.9873, 88.7539) -> (224.9748, 90.464)
  line L1034 (218.5338, 82.6214) -> (218.559, 79.1574)
  line L1035 (215.0129, 85.1927) -> (218.0254, 83.4826)
  line L1036 (224.9748, 90.464) -> (221.9875, 88.7102)
  line L1037 (214.9877, 88.6567) -> (215.0129, 85.1927)
  line L1038 (228.5714, 77.5007) -> (231.5587, 79.2545)
  line L1039 (225.5336, 82.6749) -> (225.5588, 79.2108)
  line L1040 (228.5209, 84.4287) -> (225.5336, 82.6749)
  line L1041 (220.9875, 88.7005) -> (217.975, 90.4106)
  line L1042 (221.5716, 77.4473) -> (224.5589, 79.2011)
  line L1043 (224.5337, 82.6652) -> (221.5211, 84.3753)
  line L1044 (221.9875, 88.7102) -> (222.0127, 85.2461)
  line L1045 (218.0254, 83.4826) -> (221.0127, 85.2364)
  line L1046 (225.5588, 79.2108) -> (228.5714, 77.5007)
  line L1047 (221.5211, 84.3753) -> (218.5338, 82.6214)
  line L1048 (222.0127, 85.2461) -> (225.0252, 83.536)
  line L1049 (225.0252, 83.536) -> (228.0125, 85.2898)
  line L1050 (221.0127, 85.2364) -> (220.9875, 88.7005)
  line L1051 (217.975, 90.4106) -> (214.9877, 88.6567)
  line L1052 (218.559, 79.1574) -> (221.5716, 77.4473)
  line L1053 (228.0125, 85.2898) -> (227.9873, 88.7539)
  line L1054 (231.5587, 79.2545) -> (231.5335, 82.7186)
  line L1055 (231.5335, 82.7186) -> (228.5209, 84.4287)
  line L1056 (140.5589, 91.2011) -> (140.5337, 94.6652)
  line L1057 (140.9748, 102.464) -> (137.9875, 100.7102)
  line L1058 (144.5714, 89.5007) -> (147.5587, 91.2545)
  line L1059 (141.5336, 94.6749) -> (141.5588, 91.2108)
  line L1060 (144.5209, 96.4287) -> (141.5336, 94.6749)
  line L1061 (137.5716, 89.4473) -> (140.5589, 91.2011)
  line L1062 (140.5337, 94.6652) -> (137.5211, 96.3753)
  line L1063 (141.0252, 95.536) -> (144.0125, 97.2898)
  line L1064 (134.559, 91.1574) -> (137.5716, 89.4473)
  line L1065 (147.5587, 91.2545) -> (147.5335, 94.7186)
  line L1066 (147.5335, 94.7186) -> (144.5209, 96.4287)
  line L1067 (154.5589, 91.2011) -> (154.5337, 94.6652)
  line L1068 (157.9873, 100.7539) -> (154.9748, 102.464)
  line L1069 (148.5338, 94.6214) -> (148.559, 91.1574)
  line L1070 (145.0129, 97.1927) -> (148.0254, 95.4826)
  line L1071 (154.9748, 102.464) -> (151.9875, 100.7102)
  line L1072 (144.9877, 100.6567) -> (145.0129, 97.1927)
  line L1073 (158.5714, 89.5007) -> (161.5587, 91.2545)
  line L1074 (155.5336, 94.6749) -> (155.5588, 91.2108)
  line L1075 (158.5209, 96.4287) -> (155.5336, 94.6749)
  line L1076 (151.5716, 89.4473) -> (154.5589, 91.2011)
  line L1077 (154.5337, 94.6652) -> (151.5211, 96.3753)
  line L1078 (151.9875, 100.7102) -> (152.0127, 97.2461)
  line L1079 (148.0254, 95.4826) -> (151.0127, 97.2364)
  line L1080 (155.5588, 91.2108) -> (158.5714, 89.5007)
  line L1081 (151.5211, 96.3753) -> (148.5338, 94.6214)
  line L1082 (152.0127, 97.2461) -> (155.0252, 95.536)
  line L1083 (155.0252, 95.536) -> (158.0125, 97.2898)
  line L1084 (151.0127, 97.2364) -> (150.9875, 100.7005)
  line L1085 (147.975, 102.4106) -> (144.9877, 100.6567)
  line L1086 (148.559, 91.1574) -> (151.5716, 89.4473)
  line L1087 (158.0125, 97.2898) -> (157.9873, 100.7539)
  line L1088 (161.5587, 91.2545) -> (161.5335, 94.7186)
  line L1089 (161.5335, 94.7186) -> (158.5209, 96.4287)
  line L1090 (168.5589, 91.2011) -> (168.5337, 94.6652)
  line L1091 (171.9873, 100.7539) -> (168.9748, 102.464)
  line L1092 (162.5338, 94.6214) -> (162.559, 91.1574)
  line L1093 (159.0129, 97.1927) -> (162.0254, 95.4826)
  line L1094 (168.9748, 102.464) -> (165.9875, 100.7102)
  line L1095 (158.9877, 100.6567) -> (159.0129, 97.1927)
  line L1096 (172.5714, 89.5007) -> (175.5587, 91.2545)
  line L1097 (169.5336, 94.6749) -> (169.5588, 91.2108)
  line L1098 (172.5209, 96.4287) -> (169.5336, 94.6749)
  line L1099 (164.9875, 100.7005) -> (161.975, 102.4106)
  line L1100 (165.5716, 89.4473) -> (168.5589, 91.2011)
  line L1101 (168.5337, 94.6652) -> (165.5211, 96.3753)
  line L1102 (165.9875, 100.7102) -> (166.0127, 97.2461)
  line L1103 (162.0254, 95.4826) -> (165.0127, 97.2364)
  line L1104 (169.5588, 91.2108) -> (172.5714, 89.5007)
  line L1105 (165.5211, 96.3753) -> (162.5338, 94.6214)
  line L1106 (166.0127, 97.2461) -> (169.0252, 95.536)
  line L1107 (169.0252, 95.536) -> (172.0125, 97.2898)
  line L1108 (165.0127, 97.2364) -> (164.9875, 100.7005)
  line L1109 (161.975, 102.4106) -> (158.9877, 100.6567)
  line L1110 (162.559, 91.1574) -> (165.5716, 89.4473)
  line L1111 (172.0125, 97.2898) -> (171.9873, 100.7539)
  line L1112 (175.5587, 91.2545) -> (175.5335, 94.7186)
  line L1113 (175.5335, 94.7186) -> (172.5209, 96.4287)
  line L1114 (182.5589, 91.2011) -> (182.5337, 94.6652)
  line L1115 (185.9873, 100.7539) -> (182.9748, 102.464)
  line L1116 (176.5338, 94.6214) -> (176.559, 91.1574)
  line L1117 (173.0129, 97.1927) -> (176.0254, 95.4826)
  line L1118 (182.9748, 102.464) -> (179.9875, 100.7102)
  line L1119 (172.9877, 100.6567) -> (173.0129, 97.1927)
  line L1120 (186.5714, 89.5007) -> (189.5587, 91.2545)
  line L1121 (183.5336, 94.6749) -> (183.5588, 91.2108)
  line L1122 (186.5209, 96.4287) -> (183.5336, 94.6749)
  line L1123 (178.9875, 100.7005) -> (175.975, 102.4106)
  line L1124 (179.5716, 89.4473) -> (182.5589, 91.2011)
  line L1125 (182.5337, 94.6652) -> (179.5211, 96.3753)
  line L1126 (179.9875, 100.7102) -> (180.0127, 97.2461)
  line L1127 (176.0254, 95.4826) -> (179.0127, 97.2364)
  line L1128 (183.5588, 91.2108) -> (186.5714, 89.5007)
  line L1129 (179.5211, 96.3753) -> (176.5338, 94.6214)
  line L1130 (180.0127, 97.2461) -> (183.0252, 95.536)
  line L1131 (183.0252, 95.536) -> (186.0125, 97.2898)
  line L1132 (179.0127, 97.2364) -> (178.9875, 100.7005)
  line L1133 (175.975, 102.4106) -> (172.9877, 100.6567)
  line L1134 (176.559, 91.1574) -> (179.5716, 89.4473)
  line L1135 (186.0125, 97.2898) -> (185.9873, 100.7539)
  line L1136 (189.5587, 91.2545) -> (189.5335, 94.7186)
  line L1137 (189.5335, 94.7186) -> (186.5209, 96.4287)
  line L1138 (196.5589, 91.2011) -> (196.5337, 94.6652)
  line L1139 (199.9873, 100.7539) -> (196.9748, 102.464)
  line L1140 (190.5338, 94.6214) -> (190.559, 91.1574)
  line L1141 (187.0129, 97.1927) -> (190.0254, 95.4826)
  line L1142 (196.9748, 102.464) -> (193.9875, 100.7102)
  line L1143 (186.9877, 100.6567) -> (187.0129, 97.1927)
  line L1144 (200.5714, 89.5007) -> (203.5587, 91.2545)
  line L1145 (197.5336, 94.6749) -> (197.5588, 91.2108)
  line L1146 (200.5209, 96.4287) -> (197.5336, 94.6749)
  line L1147 (192.9875, 100.7005) -> (189.975, 102.4106)
  line L1148 (193.5716, 89.4473) -> (196.5589, 91.2011)
  line L1149 (196.5337, 94.6652) -> (193.5211, 96.3753)
  line L1150 (193.9875, 100.7102) -> (194.0127, 97.2461)
  line L1151 (190.0254, 95.4826) -> (193.0127, 97.2364)
  line L1152 (197.5588, 91.2108) -> (200.5714, 89.5007)
  line L1153 (193.5211, 96.3753) -> (190.5338, 94.6214)
  line L1154 (194.0127, 97.2461) -> (197.0252, 95.536)
  line L1155 (197.0252, 95.536) -> (200.0125, 97.2898)
  line L1156 (193.0127, 97.2364) -> (192.9875, 100.7005)
  line L1157 (189.975, 102.4106) -> (186.9877, 100.6567)
  line L1158 (190.559, 91.1574) -> (193.5716, 89.4473)
  line L1159 (200.0125, 97.2898) -> (199.9873, 100.7539)
  line L1160 (203.5587, 91.2545) -> (203.5335, 94.7186)
  line L1161 (203.5335, 94.7186) -> (200.5209, 96.4287)
  line L1162 (210.5589, 91.2011) -> (210.5337, 94.6652)
  line L1163 (213.9873, 100.7539) -> (210.9748, 102.464)
  line L1164 (204.5338, 94.6214) -> (204.559, 91.1574)
  line L1165 (201.0129, 97.1927) -> (204.0254, 95.4826)
  line L1166 (210.9748, 102.464) -> (207.9875, 100.7102)
  line L1167 (200.9877, 100.6567) -> (201.0129, 97.1927)
  line L1168 (214.5714, 89.5007) -> (217.5587, 91.2545)
  line L1169 (211.5336, 94.6749) -> (211.5588, 91.2108)
  line L1170 (214.5209, 96.4287) -> (211.5336, 94.6749)
  line L1171 (206.9875, 100.7005) -> (203.975, 102.4106)
  line L1172 (207.5716, 89.4473) -> (210.5589, 91.2011)
  line L1173 (210.5337, 94.6652) -> (207.5211, 96.3753)
  line L1174 (207.9875, 100.7102) -> (208.0127, 97.2461)
  line L1175 (204.0254, 95.4826) -> (207.0127, 97.2364)
  line L1176 (211.5588, 91.2108) -> (214.5714, 89.5007)
  line L1177 (207.5211, 96.3753) -> (204.5338, 94.6214)
  line L1178 (208.0127, 97.2461) -> (211.0252, 95.536)
  line L1179 (211.0252, 95.536) -> (214.0125, 97.2898)
  line L1180 (207.0127, 97.2364) -> (206.9875, 100.7005)
  line L1181 (203.975, 102.4106) -> (200.9877, 100.6567)
  line L1182 (204.559, 91.1574) -> (207.5716, 89.4473)
  line L1183 (214.0125, 97.2898) -> (213.9873, 100.7539)
  line L1184 (217.5587, 91.2545) -> (217.5335, 94.7186)
  line L1185 (217.5335, 94.7186) -> (214.5209, 96.4287)
  line L1186 (224.5589, 91.2011) -> (224.5337, 94.6652)
  line L1187 (227.9873, 100.7539) -> (224.9748, 102.464)
  line L1188 (218.5338, 94.6214) -> (218.559, 91.1574)
  line L1189 (215.0129, 97.1927) -> (218.0254, 95.4826)
  line L1190 (224.9748, 102.464) -> (221.9875, 100.7102)
  line L1191 (214.9877, 100.6567) -> (215.0129, 97.1927)
  line L1192 (228.5714, 89.5007) -> (231.5587, 91.2545)
  line L1193 (225.5336, 94.6749) -> (225.5588, 91.2108)
  line L1194 (228.5209, 96.4287) -> (225.5336, 94.6749)
  line L1195 (220.9875, 100.7005) -> (217.975, 102.4106)
  line L1196 (221.5716, 89.4473) -> (224.5589, 91.2011)
  line L1197 (224.5337, 94.6652) -> (221.5211, 96.3753)
  line L1198 (221.9875, 100.7102) -> (222.0127, 97.2461)
  line L1199 (218.0254, 95.4826) -> (221.0127, 97.2364)
  line L1200 (225.5588, 91.2108) -> (228.5714, 89.5007)
  line L1201 (221.5211, 96.3753) -> (218.5338, 94.6214)
  line L1202 (222.0127, 97.2461) -> (225.0252, 95.536)
  line L1203 (225.0252, 95.536) -> (228.0125, 97.2898)
  line L1204 (221.0127, 97.2364) -> (220.9875, 100.7005)
  line L1205 (217.975, 102.4106) -> (214.9877, 100.6567)
  line L1206 (218.559, 91.1574) -> (221.5716, 89.4473)
  line L1207 (228.0125, 97.2898) -> (227.9873, 100.7539)
  line L1208 (231.5587, 91.2545) -> (231.5335, 94.7186)
  line L1209 (231.5335, 94.7186) -> (228.5209, 96.4287)
  point P0 (123, 72.1875)
  point P1 (137.0625, 120)
  point P2 (137.0625, 123)
  point P3 (228.9375, 6)
  point P4 (210.5625, 6)
  point P5 (183, 63)
  point P6 (176.0002, 62.9466)
  point P7 (179.5464, 56.9113)
  point P8 (186.5461, 56.9647)
  point P9 (134.0002, 26.9466)
  point P10 (144.5461, 20.9647)
  point P11 (137.5464, 20.9113)
  point P12 (141, 27)
  point P13 (141, 27)
  point P14 (141, 27)
  point P15 (148.0002, 26.9466)
  point P16 (158.5461, 20.9647)
  point P17 (151.5464, 20.9113)
  point P18 (155, 27)
  point P19 (155, 27)
  point P20 (155, 27)
  point P21 (162.0002, 26.9466)
  point P22 (172.5461, 20.9647)
  point P23 (165.5464, 20.9113)
  point P24 (169, 27)
  point P25 (169, 27)
  point P26 (169, 27)
  point P27 (176.0002, 26.9466)
  point P28 (186.5461, 20.9647)
  point P29 (179.5464, 20.9113)
  point P30 (183, 27)
  point P31 (183, 27)
  point P32 (183, 27)
  point P33 (190.0002, 26.9466)
  point P34 (200.5461, 20.9647)
  point P35 (193.5464, 20.9113)
  point P36 (197, 27)
  point P37 (197, 27)
  point P38 (197, 27)
  point P39 (204.0002, 26.9466)
  point P40 (214.5461, 20.9647)
  point P41 (207.5464, 20.9113)
  point P42 (211, 27)
  point P43 (211, 27)
  point P44 (211, 27)
  point P45 (218.0002, 26.9466)
  point P46 (228.5461, 20.9647)
  point P47 (221.5464, 20.9113)
  point P48 (225, 27)
  point P49 (225, 27)
  point P50 (225, 27)
  point P51 (134.0002, 38.9466)
  point P52 (144.5461, 32.9647)
  point P53 (137.5464, 32.9113)
  point P54 (141, 39)
  point P55 (141, 39)
  point P56 (141, 39)
  point P57 (148.0002, 38.9466)
  point P58 (158.5461, 32.9647)
  point P59 (151.5464, 32.9113)
  point P60 (155, 39)
  point P61 (155, 39)
  point P62 (155, 39)
  point P63 (162.0002, 38.9466)
  point P64 (172.5461, 32.9647)
  point P65 (165.5464, 32.9113)
  point P66 (169, 39)
  point P67 (169, 39)
  point P68 (169, 39)
  point P69 (176.0002, 38.9466)
  point P70 (186.5461, 32.9647)
  point P71 (179.5464, 32.9113)
  point P72 (183, 39)
  point P73 (183, 39)
  point P74 (183, 39)
  point P75 (190.0002, 38.9466)
  point P76 (200.5461, 32.9647)
  point P77 (193.5464, 32.9113)
  point P78 (197, 39)
  point P79 (197, 39)
  point P80 (197, 39)
  point P81 (204.0002, 38.9466)
  point P82 (214.5461, 32.9647)
  point P83 (207.5464, 32.9113)
  point P84 (211, 39)
  point P85 (211, 39)
  point P86 (211, 39)
  point P87 (218.0002, 38.9466)
  point P88 (228.5461, 32.9647)
  point P89 (221.5464, 32.9113)
  point P90 (225, 39)
  point P91 (225, 39)
  point P92 (225, 39)
  point P93 (134.0002, 50.9466)
  point P94 (144.5461, 44.9647)
  point P95 (137.5464, 44.9113)
  point P96 (141, 51)
  point P97 (141, 51)
  point P98 (141, 51)
  point P99 (148.0002, 50.9466)
  point P100 (158.5461, 44.9647)
  point P101 (151.5464, 44.9113)
  point P102 (155, 51)
  point P103 (155, 51)
  point P104 (155, 51)
  point P105 (162.0002, 50.9466)
  point P106 (172.5461, 44.9647)
  point P107 (165.5464, 44.9113)
  point P108 (169, 51)
  point P109 (169, 51)
  point P110 (169, 51)
  point P111 (176.0002, 50.9466)
  point P112 (186.5461, 44.9647)
  point P113 (179.5464, 44.9113)
  point P114 (183, 51)
  point P115 (183, 51)
  point P116 (183, 51)
  point P117 (190.0002, 50.9466)
  point P118 (200.5461, 44.9647)
  point P119 (193.5464, 44.9113)
  point P120 (197, 51)
  point P121 (197, 51)
  point P122 (197, 51)
  point P123 (204.0002, 50.9466)
  point P124 (214.5461, 44.9647)
  point P125 (207.5464, 44.9113)
  point P126 (211, 51)
  point P127 (211, 51)